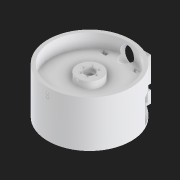
# Autodesk Inventor part: AA035c
Saved by Autodesk Inventor 2017 SP1 (Build 210196100, 196)
## iProperties
Created: 2018-03-20
Part Number: AA035c
Material: ABS Plastic
Document SubType Name: Modeling
Designer: Zach
Density: 1.06 g/cm^3
Appearance: CR White
Author: Zach
Autodesk Inventor part; units mm, degrees
ref_plane "YZ Plane" through (0, 0, 0) normal (1, 0, 0) x (0, 1, 0)
ref_plane "XZ Plane" through (0, 0, 0) normal (0, 1, 0) x (-1, 0, 0)
ref_plane "XY Plane" through (0, 0, 0) normal (0, 0, 1) x (1, 0, 0)
sketch "Sketch1" plane through (0, 0, 0) normal (0, 0, 1) x (1, 0, 0)
  circle A0 centre (0, 0) radius 60
  circle A1 centre (0, 0) radius 5
  dimension "d0" = 120
  dimension "d1" = 10
  constraints: 2 centre point, 2 coincident
  measures "d0" diameter of A0
  measures "d1" diameter of A1
extrude "Extrusion1" add sketch "Sketch1" along normal blind 67 contours A0 | A1
sketch "Sketch2" plane through (0, 0, 0) normal (0, 1, 0) x (-1, 0, 0)
  line L0 (-60, 0) -> (60, 0) projected
  line L1 (27.5, 0) -> (-27.5, 0)
  line L2 (-27.5, 0) -> (-27.5, 61)
  line L3 (-27.5, 61) -> (27.5, 61)
  line L4 (27.5, 61) -> (27.5, 0)
  point P0 (0, 0)
  point P1 (0, 0)
  dimension "d4" = 55
  dimension "d5" = 61
  constraints: 8 end point, 2 midpoint, 2 parallel, 1 horizontal, 1 perpendicular, 1 point on line
  measures "d4" distance of L2.end L3.end
  measures "d5" distance of L1.end L2.end
extrude "Extrusion2" add sketch "Sketch2" along normal blind 61.3268
sketch "Sketch3" plane through (0, 61.3268, 0) normal (0, 1, 0) x (1, 0, 0)
  line L0 (22.5, -3.5) -> (-22.5, -3.5) construction
  line L1 (-22.5, -3.5) -> (-22.5, -43.5) construction
  line L2 (-22.5, -43.5) -> (22.5, -43.5) construction
  line L3 (22.5, -43.5) -> (22.5, -3.5) construction
  line L4 (27.5, 0) -> (-27.5, 0) construction
  circle A0 centre (-22.5, -43.5) radius 2.5
  circle A1 centre (-22.5, -3.5) radius 2.5
  circle A2 centre (22.5, -3.5) radius 2.5
  circle A3 centre (22.5, -43.5) radius 2.5
  point P0 (0, 0)
  point P1 (0, -3.5)
  point P2 (0, 0)
  dimension "d8" = 45
  dimension "d9" = 40
  dimension "d10" = 3.5
  dimension "d11" = 5
  dimension "d12" = 5
  dimension "d13" = 5
  dimension "d14" = 5
  constraints: 8 end point, 4 centre point, 4 coincident, 2 midpoint, 2 parallel, 1 horizontal, 1 perpendicular, 1 vertical alignment
  measures "d8" distance of L2.end L1.end
  measures "d9" distance of L1.end L0.end
  measures "d10" distance from line of L4 L0.end
  measures "d11" diameter of A0
  measures "d12" diameter of A1
  measures "d13" diameter of A2
  measures "d14" diameter of A3
extrude "Extrusion3" cut sketch "Sketch3" against normal blind 30
sketch "Sketch4" plane through (0, 0, 67) normal (0, 0, 1) x (1, 0, 0)
  circle A0 centre (0, 0) radius 55
  dimension "d17" = 110
  constraints: 1 centre point, 1 coincident
  measures "d17" diameter of A0
extrude "Extrusion4" cut sketch "Sketch4" against normal blind 20
sketch "Sketch5" plane through (0, 0, 47) normal (0, 0, 1) x (1, 0, 0)
  circle A0 centre (0, 0) radius 17.5
  dimension "d20" = 35
  constraints: 1 centre point, 1 coincident
  measures "d20" diameter of A0
extrude "Extrusion5" add sketch "Sketch5" along normal blind 10
sketch "Sketch6" plane through (0, 0, 57) normal (0, 0, 1) x (1, 0, 0)
  circle A0 centre (0, 0) radius 5
  dimension "d23" = 10
  constraints: 1 centre point, 1 coincident
  measures "d23" diameter of A0
extrude "Extrusion6" cut sketch "Sketch6" against normal through all
sketch "Sketch7" plane through (0, 0, 57) normal (0, 0, 1) x (1, 0, 0)
  circle A0 centre (0, 0) radius 7.5
  dimension "d26" = 15
  constraints: 1 centre point, 1 coincident
  measures "d26" diameter of A0
extrude "Extrusion7" cut sketch "Sketch7" against normal blind 5
sketch "Sketch8" plane through (0, 0, 57) normal (0, 0, 1) x (1, 0, 0)
  circle A0 centre (-9.525, 0) radius 1.5
  circle A1 centre (-4.7625, -8.2489) radius 1.5
  circle A2 centre (4.7625, -8.2489) radius 1.5
  circle A3 centre (9.525, 0) radius 1.5
  circle A4 centre (4.7625, 8.2489) radius 1.5
  circle A5 centre (-4.7625, 8.2489) radius 1.5
  point P0 (0, 0)
  dimension "d29" = 3
  dimension "d30" = 9.525
  dimension "d33" = 360
  constraints: 6 centre point, 1 horizontal alignment, 13 other
  measures "d29" diameter of A0
  measures "d30" distance of point (0, 0) A0.centre
extrude "Extrusion8" cut sketch "Sketch8" against normal blind 15
sketch "Sketch9" plane through (0, 0, 0) normal (0, 1, 0) x (-1, 0, 0)
  line L0 (-7.5, 57) -> (7.5, 57) projected
  circle A0 centre (0, 54.65) radius 1.5
  circle A1 centre (0, 59.75) radius 1.5
  line L1 (0, 59.75) -> (0, 54.65)
  line L2 (0, 58.25) -> (0, 56.15)
  point P0 (0, 0)
  point P1 (0, 57.2)
  point P2 (0, 57)
  dimension "d41" = 3
  dimension "d42" = 3
  dimension "d44" = 2.1
  dimension "d45" = 1.25
  constraints: 4 end point, 3 vertical alignment, 2 midpoint, 2 point on line, 1 vertical, 4 other
  measures "d44" distance of L2.start L2.end
  measures "d45" distance from line of L0 L2.start
extrude "Extrusion9" cut sketch "Sketch9" against normal through all
sketch "Sketch10" plane through (0, 0, 0) normal (0, 0, -1) x (-1, 0, 0)
  line L0 (0, 0) -> (-33.8074, -9.0587) construction
  line L1 (0, 0) -> (35, 0) construction
  circle A0 centre (-33.8074, -9.0587) radius 2.5
  circle A1 centre (-24.7487, 24.7487) radius 2.5
  circle A2 centre (9.0587, 33.8074) radius 2.5
  circle A3 centre (33.8074, 9.0587) radius 2.5
  circle A4 centre (24.7487, -24.7487) radius 2.5
  circle A5 centre (-9.0587, -33.8074) radius 2.5
  dimension "d48" = 35
  dimension "d49" = 165
  dimension "d50" = 5
  dimension "d53" = 360
  constraints: 6 centre point, 4 end point, 3 coincident, 1 equal length, 1 horizontal, 16 other
  measures "d48" distance of L0.start L0.end
  measures "d49" angle of L0 L1
  measures "d50" diameter of A0
extrude "Extrusion10" cut sketch "Sketch10" against normal blind 25
sketch "Sketch11" plane through (0, 0, 47) normal (0, 0, 1) x (1, 0, 0)
  line L0 (-25, 31.3268) -> (-20, 31.3268) projected
  line L1 (-25, 61.3268) -> (-20, 61.3268) projected
  line L2 (20, 31.3268) -> (25, 31.3268) projected
  line L3 (20, 61.3268) -> (25, 61.3268) projected
  line L4 (27, 41.3268) -> (18, 41.3268)
  line L5 (18, 41.3268) -> (18, 46.3268)
  line L6 (18, 46.3268) -> (27, 46.3268)
  line L7 (27, 46.3268) -> (27, 41.3268)
  line L8 (-18, 41.3268) -> (-27, 41.3268)
  line L9 (-27, 41.3268) -> (-27, 46.3268)
  line L10 (-27, 46.3268) -> (-18, 46.3268)
  line L11 (-18, 46.3268) -> (-18, 41.3268)
  point P0 (0, 0)
  point P1 (-22.5, 41.3268)
  point P2 (-22.5, 31.3268)
  point P3 (22.5, 41.3268)
  point P4 (22.5, 31.3268)
  dimension "d57" = 9
  dimension "d58" = 5
  dimension "d59" = 9
  dimension "d60" = 5
  dimension "d61" = 10
  constraints: 16 end point, 4 midpoint, 4 parallel, 2 horizontal, 2 perpendicular, 2 vertical alignment, 1 horizontal alignment
  measures "d57" distance of L5.end L6.end
  measures "d58" distance of L4.end L5.end
  measures "d59" distance of L9.end L10.end
  measures "d60" distance of L8.end L9.end
  measures "d61" distance between parallel lines of L2 L4
extrude "Extrusion11" cut sketch "Sketch11" against normal blind 8.5
sketch "Sketch12" plane through (0, 0, 0) normal (0, 0, -1) x (-1, 0, 0)
  line L0 (-27, 41.3268) -> (-18, 41.3268) projected
  line L1 (-27, 46.3268) -> (-27, 41.3268) projected
  line L2 (-18, 46.3268) -> (-27, 46.3268) projected
  line L3 (-18, 41.3268) -> (-18, 46.3268) projected
  line L4 (18, 41.3268) -> (27, 41.3268) projected
  line L5 (18, 46.3268) -> (18, 41.3268) projected
  line L6 (27, 46.3268) -> (18, 46.3268) projected
  line L7 (27, 41.3268) -> (27, 46.3268) projected
  point P0 (0, 0)
extrude "Extrusion12" cut sketch "Sketch12" against normal blind 8.5
sketch "Sketch14" plane through (0, 61.3268, 0) normal (0, 1, 0) x (1, 0, 0)
  circle A0 centre (0, -21) radius 10
  line L0 (27.5, 0) -> (-27.5, 0) projected
  point P0 (0, 0)
  point P1 (0, 0)
  dimension "d68" = 20
  dimension "d69" = 21
  constraints: 1 centre point, 1 midpoint, 1 vertical alignment
  measures "d68" diameter of A0
  measures "d69" distance of point (0, 0) A0.centre
extrude "Extrusion13" cut sketch "Sketch14" against normal blind 25
sketch "Sketch26" plane through (0, 0, 0) normal (1, 0, 0) x (0, 1, 0)
  line L0 (56.3268, 3.5) -> (26.3268, 3.5)
  line L1 (26.3268, 3.5) -> (26.3268, 38.5)
  line L2 (26.3268, 38.5) -> (56.3268, 38.5)
  line L3 (56.3268, 38.5) -> (56.3268, 3.5)
  line L4 (61.3268, 31) -> (61.3268, 11) projected
  point P0 (0, 0)
  point P1 (56.3268, 21)
  point P2 (61.3268, 21)
  dimension "d124" = 30
  dimension "d125" = 35
  dimension "d126" = 5
  constraints: 8 end point, 2 midpoint, 2 parallel, 1 horizontal, 1 horizontal alignment, 1 perpendicular
  measures "d124" distance of L1.end L2.end
  measures "d125" distance of L0.end L1.end
  measures "d126" distance between parallel lines of L4 L3
extrude "Extrusion22" cut sketch "Sketch26" against normal blind 17 and the other way blind 75
sketch "Sketch28" plane through (18, 46.3268, 0) normal (0, -1, 0) x (1, 0, 0)
  line L0 (-27, 30) -> (6, 30) construction
  line L1 (6, 30) -> (6, 12) construction
  line L2 (6, 12) -> (-27, 12) construction
  line L3 (-27, 12) -> (-27, 30) construction
  circle A0 centre (-18, 21) radius 10 construction
  circle A1 centre (-27, 30) radius 2
  circle A2 centre (6, 30) radius 2
  circle A3 centre (6, 12) radius 2
  circle A4 centre (-27, 12) radius 2
  point P0 (-18, 0)
  point P1 (-27, 21)
  dimension "d131" = 33
  dimension "d132" = 18
  dimension "d133" = 9
  dimension "d134" = 4
  dimension "d135" = 4
  dimension "d136" = 4
  dimension "d137" = 4
  constraints: 8 end point, 4 centre point, 4 coincident, 2 parallel, 1 horizontal, 1 horizontal alignment, 1 midpoint, 1 perpendicular
  measures "d131" distance of L1.end L2.end
  measures "d132" distance of L0.end L1.end
  measures "d133" distance from line of L3 A0.centre
  measures "d134" diameter of A1
  measures "d135" diameter of A2
  measures "d136" diameter of A3
  measures "d137" diameter of A4
extrude "Extrusion23" cut sketch "Sketch28" against normal through all
sketch "Sketch29" plane through (18, 46.3268, 0) normal (0, -1, 0) x (1, 0, 0)
  line L0 (-18, 25) -> (27, 25)
  line L1 (27, 25) -> (27, 17)
  line L2 (27, 17) -> (-18, 17)
  line L3 (-18, 17) -> (-18, 25)
  circle A0 centre (-18, 21) radius 10 projected
  point P0 (-18, 0)
  dimension "d140" = 45
  dimension "d141" = 8
  constraints: 8 end point, 2 coincident, 2 parallel, 1 horizontal, 1 midpoint, 1 perpendicular
  measures "d140" distance from line of L1 A0.centre
  measures "d141" distance of L0.end L1.end
extrude "Extrusion24" cut sketch "Sketch29" against normal through all contours L0 A0 L2 L3 | L0 L1 L2 A0 picked at (-14.6667, 21)
ref_plane "Work Plane5" through (-27.5, 61.3268, 61) normal (0, -0.8660254, 0.5) x (1, 0, 0)
sketch "Sketch30" plane through (-27.5, 61.3268, 61) normal (0, -0.8660254, 0.5) x (1, 0, 0)
  circle A0 centre (27.5, -12) radius 10
  line L0 (0, 0) -> (55, 0) projected
  point P0 (27.5, -83.491)
  point P1 (27.5, 0)
  dimension "d145" = 20
  dimension "d146" = 12
  constraints: 1 centre point, 1 midpoint, 1 vertical alignment
  measures "d145" diameter of A0
  measures "d146" distance from line of A0.centre L0
extrude "Extrusion25" cut sketch "Sketch30" along normal through all both and the other way through all
sketch "Sketch31" plane through (0, 61.3268, 0) normal (0, 1, 0) x (1, 0, 0)
  circle A0 centre (24, -30) radius 2 projected
  circle A1 centre (-9, -30) radius 2 projected
  circle A2 centre (-9, -12) radius 2 projected
  circle A3 centre (24, -12) radius 2 projected
  circle A4 centre (24, -30) radius 3
  circle A5 centre (-9, -30) radius 3
  circle A6 centre (-9, -12) radius 3
  circle A7 centre (24, -12) radius 3
  point P0 (0, 0)
  dimension "d149" = 6
  dimension "d150" = 6
  dimension "d151" = 6
  dimension "d152" = 6
  constraints: 4 centre point, 4 coincident
  measures "d149" diameter of A4
  measures "d150" diameter of A5
  measures "d151" diameter of A6
  measures "d152" diameter of A7
extrude "Extrusion26" cut sketch "Sketch31" against normal blind 2 contours A0 | A1 | A2 | A3 | A4 | A5 | A6 | A7
equation "\"d24\" = d23"
body "Solid1"
